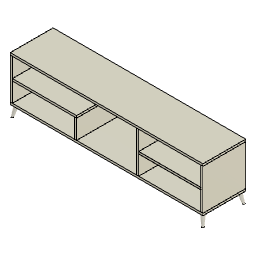
model (Autodesk Fusion 360 design; units mm, degrees)
Autodesk Fusion 360 part; units mm, degrees
ref_plane "WorkPlane1" through (0, 0, 100) normal (0, 0, 1) x (1, 0, 0)
sketch "Sketch1" plane through (0, 0, 100) normal (0, 0, 1) x (1, 0, 0)
  line L0 (0, 0) -> (1800, 0)
  line L1 (1800, 0) -> (1800, 400)
  line L2 (1800, 400) -> (0, 400)
  line L3 (0, 400) -> (0, 0)
  dimension "d2" = 1800
  dimension "d3" = 400
  constraint horizontal L0
  constraint vertical L1
  constraint horizontal L2
  constraint vertical L3
  constraint coincident L0.start L3.end
  measures "d2" distance of L0.start L0.end
  measures "d3" distance of L0.start L2.end
extrude "Extrude1" add sketch "Sketch1" along normal blind 20 makes body 1
copy_body "Body->Comp1" bodies 1 removing the originals makes body 2 in component "bottom"
sketch "Sketch2" plane through (0, 0, 120) normal (0, 0, 1) x (-1, 0, 0)
  line L0 (0, -400) -> (0, 0)
  line L1 (0, 0) -> (-1800, 0)
  line L2 (-1800, 0) -> (-1800, -400)
  line L3 (-1800, -400) -> (0, -400)
  line L4 (0, -400) -> (-20, -400)
  line L5 (-20, -400) -> (-20, 0)
  line L6 (-20, 0) -> (0, 0)
  line L7 (0, 0) -> (0, -400)
  dimension "d6" = 20
  dimension "d7" = 400
  constraint horizontal L4
  constraint vertical L5
  constraint horizontal L6
  constraint vertical L7
  constraint coincident L0.start L3.end
  measures "d6" distance of L0.start L4.end
  measures "d7" distance of L0.start L0.end
extrude "Extrude1'" add sketch "Sketch2" along normal blind 380 separate body contours L0 L1 L3 L4 L5 L6 L7 makes body 3 in component "side"
sketch "Sketch4" plane through (0, 0, 120) normal (0, 0, 1) x (-1, 0, 0)
  line L0 (0, -400) -> (0, 0)
  line L1 (0, 0) -> (-1800, 0)
  line L2 (-1800, 0) -> (-1800, -400)
  line L3 (-1800, -400) -> (0, -400)
  line L4 (0, -400) -> (-20, -400)
  line L5 (-20, -400) -> (-20, 0)
  line L6 (-20, 0) -> (0, 0)
  line L7 (0, 0) -> (0, -400)
  dimension "d11" = 20
  dimension "d12" = 400
  constraint horizontal L4
  constraint vertical L5
  constraint horizontal L6
  constraint vertical L7
  constraint coincident L0.start L3.end
  measures "d11" distance of L0.start L4.end
  measures "d12" distance of L0.start L0.end
extrude "Extrude1''" add sketch "Sketch4" along normal blind 180 separate body contours L0 L1 L3 L4 L5 L6 L7 makes body 4 in component "half vert"
sketch "Sketch5" plane through (0, 0, 300) normal (0, 0, 1) x (-1, 0, 0)
  line L0 (-20, -400) -> (-620, -400)
  line L1 (-620, -400) -> (-620, 0)
  line L2 (-620, 0) -> (-20, 0)
  line L3 (-20, 0) -> (-20, -400)
  constraint horizontal L0
  constraint vertical L1
  constraint horizontal L2
  constraint vertical L3
extrude "Extrude1'''" add sketch "Sketch5" along normal blind 20 separate body makes body 5 in component "half shelf"
sketch "Sketch6" plane through (1200, 0, 0) normal (1, 0, 0) x (0, 1, 0)
  line L0 (0, 120) -> (400, 120)
  line L1 (400, 120) -> (400, 500)
  line L2 (400, 500) -> (0, 500)
  line L3 (0, 500) -> (0, 120)
  line L4 (0, 320) -> (400, 320)
  line L5 (400, 320) -> (400, 300)
  line L6 (400, 300) -> (0, 300)
  line L7 (0, 300) -> (0, 320)
  constraint horizontal L4
  constraint vertical L5
  constraint horizontal L6
  constraint vertical L7
  constraint coincident L1 L5.end
  constraint coincident L3 L4.start
extrude "Extrude1''''" add sketch "Sketch6" along normal up to surface (580 mm away) separate body contours L1 L3 L4 L5 L6 L7 makes body 6 in component "shelf"
sketch "Sketch7" plane through (0, 0, 100) normal (0, 0, 1) x (1, 0, 0)
  circle A0 centre (30, 30) radius 20
sketch "Sketch8" plane through (0, 0, 0) normal (0, 0, 1) x (1, 0, 0)
  circle A0 centre (10, 10) radius 10
loft "Loft1" add profiles "Sketch7", "Sketch8" section 1 section 2 separate body makes body 7
copy_body "Body->Comp3" bodies 7 removing the originals makes body 8 in component "leg"
ref_plane "WorkPlane2" through (900, 200, 310) normal (1, 0, 0) x (0, 1, 0)
ref_plane "WorkPlane3" through (900, 200, 110) normal (0, -1, 0) x (1, 0, 0)
mirror "Mirror1" about plane through (900, 200, 310) normal (1, 0, 0) of bodies 8 makes body 9 in component "leg"
mirror "Mirror2" about plane through (900, 200, 110) normal (0, -1, 0) of bodies 8 9 makes body 10 at (34.9706, 364.7356, 66.6667) makes body 11 at (1765.6386, 364.1703, 66.6667) in component "leg"
component "side" placed x (1, 0, 0) y (0, 1, 0) z (0, 0, 1) at (0, 0, 0)
component "side" placed x (1, 0, 0) y (0, 1, 0) z (0, 0, 1) at (1780, 0, 0)
component "bottom" placed x (1, 0, 0) y (0, 1, 0) z (0, 0, 1) at (0, 0, 0)
component "bottom" placed x (1, 0, 0) y (0, 1, 0) z (0, 0, 1) at (0, 0, 400)
component "side" placed x (1, 0, 0) y (0, 1, 0) z (0, 0, 1) at (1180, 0, 0)
component "half vert" placed x (1, 0, 0) y (0, 1, 0) z (0, 0, 1) at (600, 0, 0)
component "half shelf" placed x (1, 0, 0) y (0, 1, 0) z (0, 0, 1) at (0, 0, 0)
component "shelf" placed x (1, 0, 0) y (0, 1, 0) z (0, 0, 1) at (0, 0, 0)
component "leg" placed x (1, 0, 0) y (0, 1, 0) z (0, 0, 1) at (0, 0, 0)
equation "d13 = ( 380 / 2 ) * 1 mm - 10 mm"
